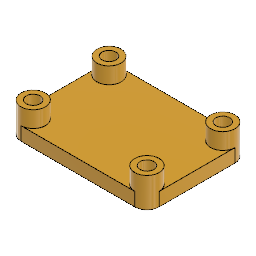
Duet3d_monitor_base v5 (Autodesk Fusion 360 design; units mm, degrees)
Autodesk Fusion 360 part; units mm, degrees
sketch "Sketch1" plane through (0, 0, 0) normal (0, 0, 1) x (1, 0, 0)
  line L0 (25.455, -18.47) -> (-25.455, -18.47)
  line L1 (-25.455, -18.47) -> (-25.455, 18.47)
  line L2 (-25.455, 18.47) -> (25.455, 18.47)
  line L3 (25.455, 18.47) -> (25.455, -18.47)
  line L4 (25.455, -18.47) -> (-25.455, 18.47) construction
  line L5 (-25.455, -18.47) -> (25.455, 18.47) construction
  circle A0 centre (20.955, 13.97) radius 4.5
  circle A1 centre (20.955, 13.97) radius 2.55
  line L6 (0, 1.75) -> (0, 22.5)
  circle A2 centre (-20.955, 13.97) radius 2.55
  circle A3 centre (-20.955, 13.97) radius 4.5
  line L7 (1.75, 0) -> (22.5, 0)
  circle A4 centre (20.955, -13.97) radius 4.5
  circle A5 centre (20.955, -13.97) radius 2.55
  circle A6 centre (-20.955, -13.97) radius 4.5
  circle A7 centre (-20.955, -13.97) radius 2.55
  dimension "d8" = 5.1
  dimension "d9" = 9
  dimension "d10" = 41.91
  dimension "d11" = 27.94
  constraint perpendicular L0 L1
  constraint parallel L0 L2
  constraint parallel L1 L3
  constraint horizontal L0
  constraint coincident L4 origin
  constraint coincident L5 origin
  constraint tangent L3 A0
  constraint tangent L2 A0
  constraint concentric A0 A1
  constraint symmetric A0 L6 A3
  constraint symmetric A1 L6 A2
  constraint symmetric A0 L7 A4
  constraint symmetric A1 L7 A5
  constraint symmetric A2 L7 A7
  constraint symmetric A3 L7 A6
  measures "d8" diameter of A1
  measures "d9" diameter of A0
  measures "d10" distance of A4.centre A6.centre
  measures "d11" distance of A0.centre A4.centre
extrude "Extrude1" add sketch "Sketch1" against normal blind 5 contours L0 L1 L2 L3 A0 A3 A4 A6 | A4 | A6 | A0 | A3 | A1 | A2 | A5 | A7
extrude "Extrude2" add sketch "Sketch1" along normal blind 6 contours A4 | A6 | A0 | A3 | A1 | A2 | A5 | A7
extrude "Extrude3" cut sketch "Sketch1" against normal blind 7 from surface at 6 contours A1 | A2 | A5 | A7
